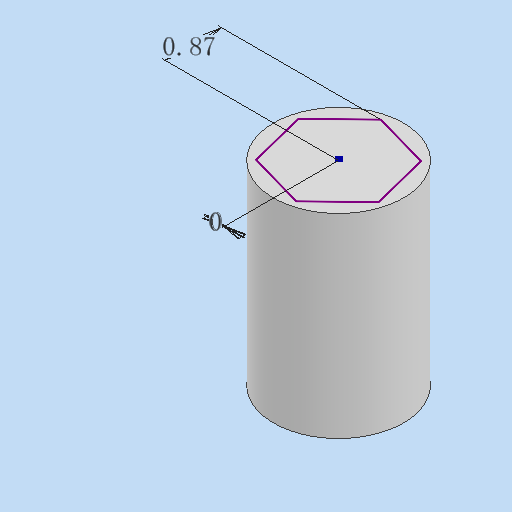
# Autodesk Inventor part: 紧定螺钉
Saved by Autodesk Inventor 2026.2 (Build 302298010, 298A)
## iProperties
Created: 2026-03-17
Part Number: 紧定螺钉
Material: 常规
Document SubType Name: Modeling
Designer: liu
Density: 1 g/cm^3
Appearance: 默认
Author: liu
Autodesk Inventor part; units mm, degrees
ref_plane "YZ Plane" through (0, 0, 0) normal (1, 0, 0) x (0, 1, 0)
ref_plane "XZ Plane" through (0, 0, 0) normal (0, 1, 0) x (-1, 0, 0)
ref_plane "XY Plane" through (0, 0, 0) normal (0, 0, 1) x (1, 0, 0)
sketch "草图1" plane through (0, 0, 0) normal (0, 1, 0) x (-1, 0, 0)
  circle A0 centre (0, 0) radius 1
  dimension "d0" = 2
  dimension "d1" = 0
  dimension "d2" = 0
  constraints: 1 centre point
  measures "d0" diameter of A0
  measures "d1" distance of point (0, 0) A0.centre
  measures "d2" distance of point (0, 0) A0.centre
extrude "拉伸1" add sketch "草图1" along normal blind 3
sketch "草图2" plane through (0, 3, 0) normal (0, 1, 0) x (1, 0, 0)
  point P0 (0, 0)
sketch "草图3" plane through (0, 3, 0) normal (0, 1, 0) x (1, 0, 0)
  line L0 (0.6435, 0.6254) -> (0.8634, -0.2446)
  line L1 (0.8634, -0.2446) -> (0.2198, -0.87)
  line L2 (0.2198, -0.87) -> (-0.6435, -0.6254)
  line L3 (-0.6435, -0.6254) -> (-0.8634, 0.2446)
  line L4 (-0.8634, 0.2446) -> (-0.2198, 0.87)
  line L5 (-0.2198, 0.87) -> (0.6435, 0.6254)
  point P0 (0, 0)
  point P1 (0, 0)
  dimension "d5" = 0.87
  dimension "d6" = 0
  dimension "d7" = 0
  constraints: 12 end point, 13 other
  measures "d5" vertical distance of L4.end point (0, 0)
  measures "d6" distance of point (0, 0) point (0, 0)
  measures "d7" distance of point (0, 0) point (0, 0)
